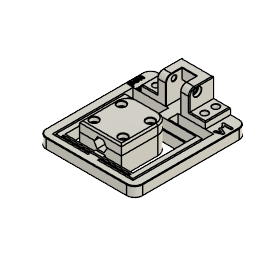
pen_mount (Autodesk Fusion 360 design; units mm, degrees)
Autodesk Fusion 360 part; units mm, degrees
sketch "Mount" plane through (0, 0, 0) normal (0, 0, 1) x (1, 0, 0) in component "Pen Mount"
  line L0 (30, -35) -> (-30, -35)
  line L1 (-30, -35) -> (-30, 35)
  line L2 (-30, 35) -> (30, 35)
  line L3 (30, 35) -> (30, -35)
  line L4 (30, -35) -> (-30, 35) construction
  line L5 (-30, -35) -> (30, 35) construction
  line L6 (25, 19) -> (25, -31)
  line L7 (-25, -31) -> (-25, 19)
  line L8 (0, 19) -> (0, -31) construction
  line L9 (0, 35) -> (0, -35) construction
  line L10 (24, 13) -> (24, -30)
  line L11 (-24, -30) -> (-24, 13)
  line L12 (-21, 12.2) -> (21, 12.2)
  line L13 (21, -29.2) -> (-21, -29.2)
  line L14 (-3, 13) -> (-3, 19)
  line L15 (3, 13) -> (3, 19)
  line L16 (-3, -30) -> (-3, -31)
  line L17 (3, -30) -> (3, -31)
  line L18 (24, -30) -> (3, -30)
  line L19 (-3, -30) -> (-24, -30)
  line L20 (-24, 13) -> (-3, 13)
  line L21 (3, 13) -> (24, 13)
  line L22 (-21, -27.2) -> (-3, -27.2)
  line L23 (-3, -27.2) -> (-3, -26.2)
  line L24 (-3, -26.2) -> (-13, -26.2)
  line L25 (-13, -26.2) -> (-13, -3.6)
  line L26 (-6, 3.4) -> (-3, 3.4)
  line L27 (-3, 3.4) -> (-3, 5.4)
  line L28 (-3, 5.4) -> (-21, 5.4)
  line L29 (-21, -28.2) -> (0, -28.2)
  line L30 (-21, 6.2) -> (0, 6.2)
  line L31 (-21, 6.2) -> (-21, 12.2)
  line L32 (-21, -29.2) -> (-21, -28.2)
  line L33 (-21, -27.2) -> (-21, 5.4)
  line L34 (21, 6.2) -> (21, 12.2)
  line L35 (21, 6.2) -> (0, 6.2)
  line L36 (3, 5.4) -> (21, 5.4)
  line L37 (3, 3.4) -> (3, 5.4)
  line L38 (6, 3.4) -> (3, 3.4)
  line L39 (13, -26.2) -> (13, -3.6)
  line L40 (21, -27.2) -> (21, 5.4)
  line L41 (3, -26.2) -> (13, -26.2)
  line L42 (3, -27.2) -> (3, -26.2)
  line L43 (21, -27.2) -> (3, -27.2)
  line L44 (21, -28.2) -> (0, -28.2)
  line L45 (21, -29.2) -> (21, -28.2)
  line L46 (-25, 19) -> (-3, 19)
  line L47 (3, 19) -> (25, 19)
  line L48 (25, -31) -> (3, -31)
  line L49 (-3, -31) -> (-25, -31)
  arc A0 (-6, 3.4) -> (-13, -3.6) centre (-6, -3.6) ccw
  arc A1 (13, -3.6) -> (6, 3.4) centre (6, -3.6) ccw
  circle A2 centre (-9, -4.2) radius 1.15
  circle A3 centre (-9, -21.2) radius 1.15
  line L50 (-9, -4.2) -> (-9, -21.2) construction
  circle A4 centre (9, -4.2) radius 1.15
  line L51 (9, -4.2) -> (9, -21.2) construction
  circle A5 centre (9, -21.2) radius 1.15
  circle A6 centre (-15, 30.5) radius 1.75
  line L52 (-15, 30.5) -> (-15, 23.5) construction
  circle A7 centre (-15, 23.5) radius 1.75
  circle A8 centre (15, 30.5) radius 1.75
  line L53 (15, 30.5) -> (15, 23.5) construction
  circle A9 centre (15, 23.5) radius 1.75
  line L54 (-4.2665, 3.4) -> (-4.2665, -26.2)
  line L55 (4.2665, 3.4) -> (4.2665, -26.2)
  line L56 (-3, 3.4) -> (3, 3.4)
  line L57 (-3, -26.2) -> (3, -26.2)
  dimension "d1" = 60
  dimension "d2" = 70
  dimension "d3" = 5
  dimension "d4" = 4
  dimension "d5" = 50
  dimension "d6" = 6
  dimension "d7" = 6
  dimension "d8" = 0.8
  dimension "d9" = 0.8
  dimension "d11" = 3
  dimension "d12" = 6
  dimension "d13" = 1
  dimension "d14" = 1
  dimension "d16" = 1
  dimension "d17" = 1
  dimension "d18" = 1
  dimension "d19" = 2
  dimension "d20" = 0.8
  dimension "d22" = 6
  dimension "d23" = 26
  dimension "d24" = 7
  dimension "d25" = 2.3
  dimension "d27" = 17
  dimension "d28" = 5
  dimension "d29" = 18
  dimension "d30" = 4
  dimension "d32" = 3.5
  dimension "d34" = 4.5
  dimension "d35" = 4.5
  dimension "d40" = 4.2665
  dimension "d73" = 30
  dimension "d74" = 7
  constraint horizontal L0
  constraint perpendicular L0 L1
  constraint parallel L0 L2
  constraint parallel L1 L3
  constraint coincident L4 origin
  constraint coincident L5 origin
  constraint horizontal L46
  constraint vertical L6
  constraint horizontal L48
  constraint vertical L7
  constraint midpoint L2 L9.start
  constraint midpoint L0 L9.end
  constraint collinear L8 L9
  constraint horizontal L20
  constraint vertical L10
  constraint horizontal L18
  constraint vertical L11
  constraint horizontal L12
  constraint horizontal L13
  constraint vertical L32
  constraint perpendicular L14 L46
  constraint symmetric L9 L14.start L15.start
  constraint symmetric L9 L14.end L15.end
  constraint coincident L16.start L18
  constraint coincident L16.end L48
  constraint perpendicular L16 L48
  constraint symmetric L9 L16.start L17.start
  constraint symmetric L9 L16.end L17.end
  constraint collinear L18 L19
  constraint collinear L20 L21
  constraint coincident L22.start L32
  constraint perpendicular L22 L32
  constraint perpendicular L22 L23
  constraint perpendicular L23 L24
  constraint perpendicular L24 L25
  constraint perpendicular L23 L26
  constraint perpendicular L26 L27
  constraint perpendicular L28 L32
  constraint horizontal L29
  constraint coincident L8 L29.end
  constraint coincident L9 L29.end
  constraint horizontal L30
  constraint coincident L30.start L32
  constraint coincident L8 L30.end
  constraint collinear L16 L23
  constraint collinear L14 L27
  constraint collinear L31 L32
  constraint collinear L32 L33
  constraint symmetric L8 L12.start L12.end
  constraint symmetric L8 L13.end L13.start
  constraint symmetric L8 L22.start L40.start
  constraint symmetric L8 L22.end L42.start
  constraint symmetric L8 L23.end L41.start
  constraint symmetric L8 L24.end L39.start
  constraint symmetric L8 L26.end L37.start
  constraint symmetric L8 L27.end L36.start
  constraint symmetric L8 L28.end L36.end
  constraint symmetric L8 L29.start L44.start
  constraint symmetric L8 L29.end L44.end
  constraint symmetric L8 L30.start L34.start
  constraint symmetric L8 L30.end L35.end
  constraint collinear L46 L47
  constraint coincident L8.start L46
  constraint collinear L48 L49
  constraint tangent L26 A0
  constraint tangent L25 A0
  constraint tangent L38 A1
  constraint tangent L39 A1
  constraint equal A0 A1
  constraint perpendicular L37 L38
  constraint equal A2 A3
  constraint coincident A2.centre L50.start
  constraint coincident A3.centre L50.end
  constraint vertical L50
  constraint symmetric L9 A2 A4
  constraint symmetric L9 A3 A5
  constraint symmetric L9 A2.centre A4.centre
  constraint symmetric L9 A3.centre L51.end
  constraint coincident L12.end L34.end
  constraint coincident L13.start L45.start
  constraint coincident A6.centre L52.start
  constraint vertical L52
  constraint coincident L52.end A7.centre
  constraint equal A6 A7
  constraint symmetric L9 A6 A8
  constraint symmetric L9 A6.centre A8.centre
  constraint symmetric L9 L52.end L53.end
  constraint symmetric L9 A7 A9
  constraint coincident L26 L54.start
  constraint coincident L24 L54.end
  constraint perpendicular L24 L54
  constraint symmetric L9 L54.start L55.start
  constraint symmetric L9 L54.end L55.end
  measures "d1" distance of L1.end L2.end
  measures "d2" distance of L0.end L1.end
  measures "d3" distance of L1 L7
  measures "d4" distance of L0 L48
  measures "d5" distance of L6.start L6.end
  measures "d6" distance of L14 L15
  measures "d7" distance of L16 L17
  measures "d8" distance of L12 L20
  measures "d9" distance of L13 L18
  measures "d11" distance of L11 L32
  measures "d12" distance of L14.start L14.end
  measures "d13" distance of L16.start L16.end
  measures "d14" distance of L7 L11
  measures "d16" distance of L13 L29
  measures "d17" distance of L22 L29
  measures "d18" distance of L22.end L23.end
  measures "d19" distance of L26.end L27.end
  measures "d20" distance of L28 L30
  measures "d22" distance of L12 L30
  measures "d23" distance of L25 L39
  measures "d24" radius of A0
  measures "d25" diameter of A2
  measures "d27" distance of A2.centre A3.centre
  measures "d28" distance of L24 A3.centre
  measures "d29" distance of L50 L51
  measures "d30" distance of L25 L50
  measures "d32" diameter of A6
  measures "d34" distance of L2 A6.centre
  measures "d35" distance of L46 L52.end
  measures "d40" distance of L9 L54
  measures "d73" distance of L52 L53
  measures "d74" distance of A6.centre L52.end
extrude "Extrude1" add sketch "Mount" along normal blind 6.5 contours L0 L1 L2 L3 | L24 L26 L38 L41 L54 L55 L56 L57 | L24 L25 L26 A0 L54 | L38 L39 L41 A1 L55 makes body 1 in component "Pen Mount"
extrude "Extrude3" add sketch "Mount" along normal blind 1 from surface at 6.5 contours L24 L26 L38 L41 L54 L55 L56 L57 | L24 L25 L26 A0 L54 | L38 L39 L41 A1 L55 bodies 1 in component "Pen Mount"
extrude "Extrude2" add sketch "Mount" along normal blind 3.695 from surface at 7.5 contours L24 L25 L26 A0 L54 | L38 L39 L41 A1 L55 bodies 1 in component "Pen Mount"
sketch "Sketch1" plane through (0, 0, 11.195) normal (0, 0, 1) x (-1, 0, 0) in component "Clamp"
  line L0 (4.2665, -3.4) -> (6, -3.4)
  arc A0 (6, -3.4) -> (13, 3.6) centre (6, 3.6) ccw
  line L1 (13, 3.6) -> (13, 26.2)
  line L2 (13, 26.2) -> (4.2665, 26.2)
  line L3 (4.2665, 26.2) -> (4.2665, -3.4)
  circle A1 centre (9, 4.2) radius 1.15
  circle A2 centre (9, 21.2) radius 1.15
  line L4 (4.2665, -3.4) -> (4.2665, 26.2)
  line L5 (4.2665, 26.2) -> (-4.2665, 26.2)
  line L6 (-4.2665, 26.2) -> (-4.2665, -3.4)
  line L7 (-4.2665, -3.4) -> (4.2665, -3.4)
  line L8 (-6, -3.4) -> (-4.2665, -3.4)
  line L9 (-4.2665, -3.4) -> (-4.2665, 26.2)
  line L10 (-4.2665, 26.2) -> (-13, 26.2)
  line L11 (-13, 26.2) -> (-13, 3.6)
  arc A3 (-13, 3.6) -> (-6, -3.4) centre (-6, 3.6) ccw
  circle A4 centre (-9, 4.2) radius 1.15
  circle A5 centre (-9, 21.2) radius 1.15
  line L12 (-3.6165, -3.4) -> (-3.6165, 26.2)
  line L13 (0, -3.4) -> (0, 26.2) construction
  line L14 (3.6165, -3.4) -> (3.6165, 26.2)
  circle A6 centre (9, 4.2) radius 1.48
  circle A7 centre (-9, 4.2) radius 1.48
  circle A8 centre (-9, 21.2) radius 1.48
  circle A9 centre (9, 21.2) radius 1.48
  dimension "d64" = 0.65
  dimension "d75" = 0.33
  constraint coincident L7 L12.start
  constraint coincident L5 L12.end
  constraint perpendicular L5 L12
  constraint midpoint L7 L13.start
  constraint midpoint L5 L13.end
  constraint symmetric L12.start L13 L14.start
  constraint symmetric L12.end L13 L14.end
  constraint concentric A4 A7
  constraint concentric A5 A8
  constraint concentric A2 A9
  constraint equal A6 A9
  constraint equal A6 A7
  constraint equal A6 A8
  measures "d64" distance of L6 L12
extrude "Extrude1'" add sketch "Sketch1" along normal blind 3 from surface at 2.995 separate body contours L5 L7 L12 L14 makes body 2 in component "Clamp"
extrude "Extrude2'" add sketch "Sketch1" along normal blind 5.995 contours L0 A0 L1 L2 L3 L4 | L3 L4 L5 L7 L14 | L5 L6 L7 L9 L12 | L6 L8 L9 L10 L11 A3 bodies 2 in component "Clamp"
draft "Draft1" angle 30 neutral plane through (0, 0, 11.195) pull (0, 0, -1) 1 faces at (3.6165, -6.4667, 12.1933) on bodies 2 in component "Clamp"
draft "Draft2" angle 30 neutral plane through (0, 0, 11.195) pull (0, 0, -1) 1 faces at (-3.6165, -6.4667, 12.1933) on bodies 2 in component "Clamp"
sketch "Sketch2" plane through (0, 0, 17.19) normal (0, 0, 1) x (-1, 0, 0) in component "Clamp"
  line L0 (13, 26.2) -> (-13, 26.2)
  line L1 (-6, -3.4) -> (6, -3.4)
  circle A0 centre (9, 21.2) radius 2.45
  circle A1 centre (9, 4.2) radius 2.45
  circle A2 centre (-9, 4.2) radius 2.45
  circle A3 centre (-9, 21.2) radius 2.45
  arc A4 (6, -3.4) -> (13, 3.6) centre (6, 3.6) ccw
  line L2 (13, 3.6) -> (13, 26.2)
  line L3 (-13, 26.2) -> (-13, 3.6)
  arc A5 (-13, 3.6) -> (-6, -3.4) centre (-6, 3.6) ccw
  circle A6 centre (9, 21.2) radius 1.48
  circle A7 centre (9, 4.2) radius 1.48
  circle A8 centre (-9, 21.2) radius 1.48
  circle A9 centre (-9, 4.2) radius 1.48
  dimension "d53" = 4.9
  constraint equal A0 A1
  constraint equal A0 A2
  constraint equal A0 A3
  constraint concentric A1 A7
  constraint concentric A2 A9
  constraint concentric A3 A8
  constraint concentric A0 A6
  measures "d53" diameter of A0
extrude "Extrude3'" cut sketch "Sketch2" against normal blind 2.65 contours A0 | A1 | A2 | A3 | A6 | A7 | A8 | A9 bodies 2 in component "Clamp"
chamfer "Chamfer1" distance 1 angle 45 6 edges at (0, 3.4, 17.19) (10.9497, 1.3497, 17.19) (13, -14.9, 17.19) (-13, -14.9, 17.19) (-10.9497, 1.3497, 17.19) (0, -26.2, 17.19) on bodies 2 in component "Clamp"
draft "Draft1'" angle 30 neutral plane through (0, 0, 11.195) pull (0, 0, 1) 1 faces at (-4.2665, -16.3333, 9.9633) on bodies 1 in component "Pen Mount"
draft "Draft2'" angle 30 neutral plane through (0, 0, 11.195) pull (0, 0, 1) 1 faces at (4.2665, -16.3333, 9.9633) on bodies 1 in component "Pen Mount"
fillet "Fillet1" radius 5 4 edges at (-30, -35, 3.25) (30, -35, 3.25) (30, 35, 3.25) (-30, 35, 3.25) on bodies 1 in component "Pen Mount"
chamfer "Chamfer1'" distance 0.3 angle 45 16 edges at (30, 0, 0) (28.5355, -33.5355, 0) (0, -35, 0) (-28.5355, -33.5355, 0) (-30, 0, 0) (-28.5355, 33.5355, 0) (0, 35, 0) (28.5355, 33.5355, 0) (30, 0, 6.5) (28.5355, 33.5355, 6.5) (0, 35, 6.5) (-28.5355, 33.5355, 6.5) (-30, 0, 6.5) (-28.5355, -33.5355, 6.5) (0, -35, 6.5) (28.5355, -33.5355, 6.5) on bodies 1 in component "Pen Mount"
sketch "Pen cross section" plane through (0, -26.2, 0) normal (0, -1, 0) x (1, 0, 0) in component "Pen Mount"
  line L0 (3, 0) -> (13, 0)
  line L1 (13, 0) -> (13, 11.195)
  line L2 (13, 11.195) -> (4.2665, 11.195)
  line L3 (4.2665, 11.195) -> (2.1332, 7.5)
  line L4 (2.1332, 7.5) -> (-2.1332, 7.5)
  line L5 (-2.1332, 7.5) -> (-4.2665, 11.195)
  line L6 (-4.2665, 11.195) -> (-13, 11.195)
  line L7 (-13, 11.195) -> (-13, 0)
  line L8 (-13, 0) -> (-3, 0)
  line L9 (-3, 0) -> (-3, 6.5)
  line L10 (-3, 6.5) -> (3, 6.5)
  line L11 (3, 6.5) -> (3, 0)
  line L12 (-2.1333, 7.5) -> (2.1333, 7.5)
  line L13 (2.1333, 7.5) -> (4.2666, 11.195)
  line L14 (4.2666, 11.195) -> (2.1333, 14.89)
  line L15 (2.1333, 14.89) -> (-2.1333, 14.89)
  line L16 (-2.1333, 14.89) -> (-4.2666, 11.195)
  line L17 (-4.2666, 11.195) -> (-2.1333, 7.5)
  line L18 (0, 14.89) -> (0, 7.5) construction
  point P0 (0, 11.195)
  dimension "d69" = 8.5332
  dimension "d70" = 7.39
  constraint collinear L4 L12
  constraint midpoint L15 L18.start
  constraint midpoint L12 L18.end
  constraint midpoint L4 L18.end
  measures "d69" distance of L13.end L16.end
  measures "d70" distance of L12 L15
fillet "Fillet1'" radius 0.5 2 edges at (-3.6165, -11.4, 11.195) (3.6165, -11.4, 11.195) on bodies 2 in component "Clamp"
sketch "Mounting screw heads" plane through (0, 0, 6.5) normal (0, 0, 1) x (-1, 0, 0) in component "Pen Mount"
  circle A0 centre (-15, -23.5) radius 1.75
  circle A1 centre (-15, -30.5) radius 1.75
  circle A2 centre (15, -23.5) radius 1.75
  circle A3 centre (15, -30.5) radius 1.75
  line L0 (-21, 29.2) -> (21, 29.2)
  line L1 (21, 29.2) -> (21, 28.2)
  line L2 (21, 28.2) -> (-21, 28.2)
  line L3 (-21, 28.2) -> (-21, 29.2)
  line L4 (-21, -6.2) -> (21, -6.2)
  line L5 (21, -6.2) -> (21, -12.2)
  line L6 (21, -12.2) -> (-21, -12.2)
  line L7 (-21, -12.2) -> (-21, -6.2)
  line L8 (24, 30) -> (3, 30)
  line L9 (3, 30) -> (3, 31)
  line L10 (3, 31) -> (25, 31)
  line L11 (25, 31) -> (25, -19)
  line L12 (25, -19) -> (3, -19)
  line L13 (3, -19) -> (3, -13)
  line L14 (3, -13) -> (24, -13)
  line L15 (24, -13) -> (24, 30)
  line L16 (-3, 26.2) -> (3, 26.2)
  line L17 (3, 26.2) -> (3, 27.2)
  line L18 (3, 27.2) -> (21, 27.2)
  line L19 (21, 27.2) -> (21, -5.4)
  line L20 (21, -5.4) -> (3, -5.4)
  line L21 (3, -5.4) -> (3, -3.4)
  line L22 (3, -3.4) -> (-3, -3.4)
  line L23 (-3, -3.4) -> (-3, -5.4)
  line L24 (-3, -5.4) -> (-21, -5.4)
  line L25 (-21, -5.4) -> (-21, 27.2)
  line L26 (-21, 27.2) -> (-3, 27.2)
  line L27 (-3, 27.2) -> (-3, 26.2)
  line L28 (-24, -13) -> (-3, -13)
  line L29 (-3, -13) -> (-3, -19)
  line L30 (-3, -19) -> (-25, -19)
  line L31 (-25, -19) -> (-25, 31)
  line L32 (-25, 31) -> (-3, 31)
  line L33 (-3, 31) -> (-3, 30)
  line L34 (-3, 30) -> (-24, 30)
  line L35 (-24, 30) -> (-24, -13)
  line L36 (29.7, -30) -> (29.7, 30)
  arc A4 (29.7, 30) -> (25, 34.7) centre (25, 30) ccw
  line L37 (25, 34.7) -> (-25, 34.7)
  arc A5 (-25, 34.7) -> (-29.7, 30) centre (-25, 30) ccw
  line L38 (-29.7, 30) -> (-29.7, -30)
  arc A6 (-29.7, -30) -> (-25, -34.7) centre (-25, -30) ccw
  line L39 (-25, -34.7) -> (25, -34.7)
  arc A7 (25, -34.7) -> (29.7, -30) centre (25, -30) ccw
  circle A8 centre (15, -30.5) radius 3
  circle A9 centre (15, -23.5) radius 3
  circle A10 centre (-15, -30.5) radius 3
  circle A11 centre (-15, -23.5) radius 3
  line L40 (-27.7, -20) -> (-27.7, -33.2) construction
  line L41 (-27.7, -33.2) -> (-22.2993, -33.2) construction
  line L42 (-22.2993, -33.2) -> (-22.2993, -20) construction
  line L43 (-22.2993, -20) -> (-27.7, -20) construction
  line L44 (24.0828, -19.2154) -> (24.0761, -31.7956) construction
  line L45 (24.0761, -31.7956) -> (29.0761, -31.7983) construction
  line L46 (29.0761, -31.7983) -> (29.0828, -19.2181) construction
  line L47 (29.0828, -19.2181) -> (24.0828, -19.2154) construction
  dimension "d76" = 6
  dimension "d87" = 6
  dimension "d88" = 1
  dimension "d89" = 1.5
  dimension "d90" = 2
  dimension "d93" = 3.7
  text T0 "v1\n" font "Arial" height 6 bold align left top in box 13.2 x 5.4007 at (-27.7, -20) x (0, -1) y (1, 0) spacing 1 kerned
  text T1 "pen\nmount" font "Arial" height 3.7 bold align left top in box 12.5802 x 5 at (24.0828, -19.2154) x (-0.000531, -1) y (1, -0.000531) spacing 1 kerned
  constraint concentric A3 A8
  constraint concentric A2 A9
  constraint concentric A1 A10
  constraint concentric A0 A11
  constraint equal A8 A9
  constraint equal A8 A10
  constraint equal A8 A11
  measures "d76" diameter of A8
  measures "d88" distance of L30 L43
  measures "d89" distance of L39 L41
  measures "d90" distance of L38 L40
fillet "Fillet2" radius 0.25 4 faces at (-13.2587, 23.3258, 4.3333) (-13.2587, 30.3258, 4.3333) (16.7413, 30.3258, 4.3333) (16.7413, 23.3258, 4.3333) on bodies 1 in component "Pen Mount"
fillet "Fillet2" radius 0.25 4 faces at (-7.8557, -4.3145, 3.7317) (-8.3287, -20.2663, 3.7317) (10.1443, -4.3145, 3.7317) (9.6713, -20.2663, 3.7317) on bodies 1 in component "Pen Mount"
fillet "Fillet2'" radius 0.25 4 edges at (-6.7158, -5.086, 17.19) (11.2842, -5.086, 17.19) (11.2842, -22.086, 17.19) (-6.7158, -22.086, 17.19) on bodies 2 in component "Clamp"
extrude "Extrude4" add sketch "Mounting screw heads" along normal blind 0.2 text T0 T1 bodies 1 in component "Pen Mount"
sketch "Sketch1 (2)" plane through (0, 0, 6.5) normal (0, 0, 1) x (-1, 0, 0) in component "Weight mount"
  spline S0 degree 3 poles (21.9429, -23.6992) (22.0605, -23.7069) (22.2992, -23.7226) (22.5165, -23.8229) (22.6268, -23.8737) knots 0 0 0 0 0.035038 0.071116 0.071116 0.071116 0.071116
  spline S1 degree 3 poles (22.6268, -23.8737) (22.7302, -23.9375) (22.9356, -24.0641) (23.0664, -24.2668) (23.1313, -24.3674) knots 0 0 0 0 0.035952 0.071388 0.071388 0.071388 0.071388
  spline S2 degree 3 poles (23.1313, -24.3674) (23.182, -24.4783) (23.2856, -24.7047) (23.2985, -24.9535) (23.3051, -25.0805) knots 0 0 0 0 0.036225 0.073988 0.073988 0.073988 0.073988
  spline S3 degree 3 poles (23.3051, -25.0805) (23.2903, -25.2723) (23.2615, -25.6461) (23.0248, -25.936) (22.9095, -26.0772) knots 0 0 0 0 0.05621 0.10955 0.10955 0.10955 0.10955
  spline S4 degree 3 poles (22.9095, -26.0772) (22.7669, -26.1905) (22.4745, -26.4225) (22.1019, -26.4509) (21.9111, -26.4654) knots 0 0 0 0 0.053369 0.109334 0.109334 0.109334 0.109334
  spline S5 degree 3 poles (21.9111, -26.4654) (21.7187, -26.4505) (21.3424, -26.4213) (21.0473, -26.1869) (20.9031, -26.0724) knots 0 0 0 0 0.056479 0.110425 0.110425 0.110425 0.110425
  spline S6 degree 3 poles (20.9031, -26.0724) (20.7865, -25.9314) (20.5492, -25.6444) (20.5189, -25.273) (20.5036, -25.0841) knots 0 0 0 0 0.053525 0.108919 0.108919 0.108919 0.108919
  spline S7 degree 3 poles (20.5036, -25.0841) (20.5107, -24.9625) (20.5249, -24.7184) (20.6219, -24.4939) (20.6705, -24.3812) knots 0 0 0 0 0.036237 0.072735 0.072735 0.072735 0.072735
  spline S8 degree 3 poles (20.6705, -24.3812) (20.7322, -24.2766) (20.8551, -24.0686) (21.0582, -23.9379) (21.1591, -23.8729) knots 0 0 0 0 0.035892 0.071384 0.071384 0.071384 0.071384
  spline S9 degree 3 poles (21.1591, -23.8729) (21.2764, -23.8223) (21.5262, -23.7144) (21.7985, -23.7045) (21.9429, -23.6992) knots 0 0 0 0 0.037997 0.080903 0.080903 0.080903 0.080903
  line L0 (23.2476, -19.215) -> (23.2473, -19.8687)
  line L1 (23.2473, -19.8687) -> (22.8813, -19.8685)
  spline S10 degree 3 poles (22.8813, -19.8685) (23.0056, -19.9878) (23.2451, -20.2177) (23.2872, -20.5461) (23.3074, -20.7041) knots 0 0 0 0 0.049999 0.096357 0.096357 0.096357 0.096357
  spline S11 degree 3 poles (23.3074, -20.7041) (23.3038, -20.7855) (23.2969, -20.9414) (23.2321, -21.0831) (23.2011, -21.1508) knots 0 0 0 0 0.024186 0.046297 0.046297 0.046297 0.046297
  spline S12 degree 3 poles (23.2011, -21.1508) (23.1601, -21.2116) (23.0752, -21.3376) (22.9468, -21.419) (22.8804, -21.461) knots 0 0 0 0 0.021771 0.045054 0.045054 0.045054 0.045054
  spline S13 degree 3 poles (22.8804, -21.461) (22.9464, -21.5193) (23.0723, -21.6305) (23.1594, -21.774) (23.2008, -21.8423) knots 0 0 0 0 0.026236 0.050053 0.050053 0.050053 0.050053
  spline S14 degree 3 poles (23.2008, -21.8423) (23.2317, -21.9117) (23.2935, -22.0508) (23.3022, -22.2028) (23.3065, -22.279) knots 0 0 0 0 0.022583 0.045264 0.045264 0.045264 0.045264
  spline S15 degree 3 poles (23.3065, -22.279) (23.3028, -22.3714) (23.2956, -22.5461) (23.2214, -22.7042) (23.1864, -22.7787) knots 0 0 0 0 0.027422 0.051852 0.051852 0.051852 0.051852
  spline S16 degree 3 poles (23.1864, -22.7787) (23.1411, -22.8428) (23.0487, -22.9733) (22.9065, -23.0466) (22.8342, -23.0839) knots 0 0 0 0 0.02319 0.047221 0.047221 0.047221 0.047221
  spline S17 degree 3 poles (22.8342, -23.0839) (22.7597, -23.105) (22.5786, -23.1564) (22.3899, -23.1566) (22.2789, -23.1568) knots 0 0 0 0 0.023124 0.056237 0.056237 0.056237 0.056237
  line L2 (22.2789, -23.1568) -> (20.5652, -23.1558)
  line L3 (20.5652, -23.1558) -> (20.5655, -22.4466)
  line L4 (20.5655, -22.4466) -> (22.0975, -22.4475)
  spline S18 degree 3 poles (22.0975, -22.4475) (22.2082, -22.4492) (22.3845, -22.452) (22.5506, -22.3955) (22.6124, -22.3745) knots 0 0 0 0 0.032861 0.052328 0.052328 0.052328 0.052328
  spline S19 degree 3 poles (22.6124, -22.3745) (22.6566, -22.3361) (22.7484, -22.2564) (22.7587, -22.1348) (22.764, -22.0717) knots 0 0 0 0 0.016884 0.035076 0.035076 0.035076 0.035076
  spline S20 degree 3 poles (22.764, -22.0717) (22.76, -22.0225) (22.7518, -21.922) (22.6998, -21.8356) (22.6733, -21.7915) knots 0 0 0 0 0.014627 0.029808 0.029808 0.029808 0.029808
  spline S21 degree 3 poles (22.6733, -21.7915) (22.6384, -21.7505) (22.5659, -21.665) (22.4614, -21.6236) (22.4071, -21.6021) knots 0 0 0 0 0.015906 0.033119 0.033119 0.033119 0.033119
  spline S22 degree 3 poles (22.4071, -21.6021) (22.332, -21.5853) (22.1499, -21.5444) (21.963, -21.544) (21.8532, -21.5438) knots 0 0 0 0 0.023035 0.055846 0.055846 0.055846 0.055846
  line L5 (21.8532, -21.5438) -> (20.566, -21.5431)
  line L6 (20.566, -21.5431) -> (20.5664, -20.8339)
  line L7 (20.5664, -20.8339) -> (22.0353, -20.8347)
  spline S23 degree 3 poles (22.0353, -20.8347) (22.1429, -20.8358) (22.3125, -20.8376) (22.4792, -20.8079) (22.5401, -20.7971) knots 0 0 0 0 0.032193 0.05071 0.05071 0.05071 0.05071
  spline S24 degree 3 poles (22.5401, -20.7971) (22.5749, -20.7836) (22.6409, -20.758) (22.6873, -20.7049) (22.7092, -20.6798) knots 0 0 0 0 0.01102 0.020858 0.020858 0.020858 0.020858
  spline S25 degree 3 poles (22.7092, -20.6798) (22.7254, -20.6492) (22.761, -20.5819) (22.7635, -20.5056) (22.7649, -20.464) knots 0 0 0 0 0.010254 0.022541 0.022541 0.022541 0.022541
  spline S26 degree 3 poles (22.7649, -20.464) (22.7614, -20.4109) (22.7544, -20.3058) (22.7024, -20.2141) (22.6767, -20.1687) knots 0 0 0 0 0.015741 0.031179 0.031179 0.031179 0.031179
  spline S27 degree 3 poles (22.6767, -20.1687) (22.6433, -20.1278) (22.5744, -20.0435) (22.4737, -20.0019) (22.4219, -19.9805) knots 0 0 0 0 0.015597 0.032119 0.032119 0.032119 0.032119
  spline S28 degree 3 poles (22.4219, -19.9805) (22.3483, -19.9641) (22.1666, -19.9234) (21.9802, -19.9234) (21.8692, -19.9235) knots 0 0 0 0 0.022553 0.055709 0.055709 0.055709 0.055709
  line L8 (21.8692, -19.9235) -> (20.5669, -19.9228)
  line L9 (20.5669, -19.9228) -> (20.5672, -19.2136)
  line L10 (20.5672, -19.2136) -> (23.2476, -19.215)
  circle A0 centre (-15, -23.5) radius 2
  circle A1 centre (15, -30.5) radius 2
  line L11 (-29.7, 30) -> (-29.7, -30)
  arc A2 (-29.7, -30) -> (-25, -34.7) centre (-25, -30) ccw
  line L12 (-25, -34.7) -> (25, -34.7)
  arc A3 (25, -34.7) -> (29.7, -30) centre (25, -30) ccw
  line L13 (29.7, -30) -> (29.7, 30)
  arc A4 (29.7, 30) -> (25, 34.7) centre (25, 30) ccw
  line L14 (25, 34.7) -> (-25, 34.7)
  arc A5 (-25, 34.7) -> (-29.7, 30) centre (-25, 30) ccw
  line L15 (-21, -6.2) -> (21, -6.2)
  line L16 (21, -6.2) -> (21, -12.2)
  line L17 (21, -12.2) -> (-21, -12.2)
  line L18 (-21, -12.2) -> (-21, -6.2)
  line L19 (-21, 29.2) -> (21, 29.2)
  line L20 (21, 29.2) -> (21, 28.2)
  line L21 (21, 28.2) -> (-21, 28.2)
  line L22 (-21, 28.2) -> (-21, 29.2)
  line L23 (-24, -13) -> (-3, -13)
  line L24 (-3, -13) -> (-3, -19)
  line L25 (-3, -19) -> (-25, -19)
  line L26 (-25, -19) -> (-25, 31)
  line L27 (-25, 31) -> (-3, 31)
  line L28 (-3, 31) -> (-3, 30)
  line L29 (-3, 30) -> (-24, 30)
  line L30 (-24, 30) -> (-24, -13)
  line L31 (24, 30) -> (3, 30)
  line L32 (3, 30) -> (3, 31)
  line L33 (3, 31) -> (25, 31)
  line L34 (25, 31) -> (25, -19)
  line L35 (25, -19) -> (3, -19)
  line L36 (3, -19) -> (3, -13)
  line L37 (3, -13) -> (24, -13)
  line L38 (24, -13) -> (24, 30)
  line L39 (-3, 26.2) -> (3, 26.2)
  line L40 (3, 26.2) -> (3, 27.2)
  line L41 (3, 27.2) -> (21, 27.2)
  line L42 (21, 27.2) -> (21, -5.4)
  line L43 (21, -5.4) -> (3, -5.4)
  line L44 (3, -5.4) -> (3, -3.4)
  line L45 (3, -3.4) -> (-3, -3.4)
  line L46 (-3, -3.4) -> (-3, -5.4)
  line L47 (-3, -5.4) -> (-21, -5.4)
  line L48 (-21, -5.4) -> (-21, 27.2)
  line L49 (-21, 27.2) -> (-3, 27.2)
  line L50 (-3, 27.2) -> (-3, 26.2)
  circle A6 centre (15, -23.5) radius 2
  circle A7 centre (-15, -30.5) radius 2
  line L51 (27.1924, -23.9796) -> (27.0734, -24.6862)
  spline S29 degree 3 poles (27.0734, -24.6862) (26.953, -24.6362) (26.7211, -24.5397) (26.5595, -24.3479) (26.4818, -24.2556) knots 0 0 0 0 0.038477 0.074127 0.074127 0.074127 0.074127
  spline S30 degree 3 poles (26.4818, -24.2556) (26.4226, -24.1477) (26.2973, -23.9189) (26.2853, -23.6577) (26.279, -23.5198) knots 0 0 0 0 0.036434 0.077228 0.077228 0.077228 0.077228
  spline S31 degree 3 poles (26.279, -23.5198) (26.293, -23.3059) (26.3194, -22.903) (26.6032, -22.6187) (26.7364, -22.4852) knots 0 0 0 0 0.061888 0.116598 0.116598 0.116598 0.116598
  spline S32 degree 3 poles (26.7364, -22.4852) (26.8711, -22.4081) (27.1568, -22.2445) (27.4862, -22.229) (27.6603, -22.2207) knots 0 0 0 0 0.045916 0.097327 0.097327 0.097327 0.097327
  spline S33 degree 3 poles (27.6603, -22.2207) (27.865, -22.2307) (28.2469, -22.2493) (28.5589, -22.4681) (28.7037, -22.5696) knots 0 0 0 0 0.06004 0.112035 0.112035 0.112035 0.112035
  spline S34 degree 3 poles (28.7037, -22.5696) (28.8137, -22.6943) (29.0359, -22.9464) (29.0656, -23.2814) (29.0805, -23.4506) knots 0 0 0 0 0.048539 0.098092 0.098092 0.098092 0.098092
  spline S35 degree 3 poles (29.0805, -23.4506) (29.0666, -23.6371) (29.0397, -23.9967) (28.8003, -24.2651) (28.6851, -24.3943) knots 0 0 0 0 0.05441 0.1049 0.1049 0.1049 0.1049
  spline S36 degree 3 poles (28.6851, -24.3943) (28.5226, -24.4938) (28.1536, -24.7199) (27.7183, -24.7227) (27.4747, -24.7243) knots 0 0 0 0 0.056156 0.127567 0.127567 0.127567 0.127567
  line L52 (27.4747, -24.7243) -> (27.4756, -22.9475)
  spline S37 degree 3 poles (27.4756, -22.9475) (27.3789, -22.9542) (27.199, -22.9667) (27.0524, -23.0707) (26.9846, -23.1189) knots 0 0 0 0 0.028433 0.052905 0.052905 0.052905 0.052905
  spline S38 degree 3 poles (26.9846, -23.1189) (26.9335, -23.1771) (26.8305, -23.2942) (26.8162, -23.4496) (26.809, -23.5276) knots 0 0 0 0 0.022639 0.045526 0.045526 0.045526 0.045526
  spline S39 degree 3 poles (26.809, -23.5276) (26.8122, -23.5802) (26.8183, -23.6816) (26.8733, -23.7668) (26.8997, -23.8078) knots 0 0 0 0 0.0155 0.029897 0.029897 0.029897 0.029897
  spline S40 degree 3 poles (26.8997, -23.8078) (26.9374, -23.8441) (27.0209, -23.9246) (27.1316, -23.9601) (27.1924, -23.9796) knots 0 0 0 0 0.015495 0.034337 0.034337 0.034337 0.034337
  line L53 (20.5601, -32.6153) -> (20.5605, -31.9061)
  line L54 (20.5605, -31.9061) -> (21.9284, -31.9068)
  spline S41 degree 3 poles (21.9284, -31.9068) (22.0481, -31.9081) (22.237, -31.9102) (22.4222, -31.8747) (22.49, -31.8617) knots 0 0 0 0 0.035762 0.056457 0.056457 0.056457 0.056457
  spline S42 degree 3 poles (22.49, -31.8617) (22.5299, -31.8446) (22.6078, -31.8112) (22.6618, -31.746) (22.6882, -31.7142) knots 0 0 0 0 0.0128 0.025026 0.025026 0.025026 0.025026
  spline S43 degree 3 poles (22.6882, -31.7142) (22.7089, -31.6775) (22.7518, -31.6012) (22.7566, -31.5136) (22.759, -31.4681) knots 0 0 0 0 0.012448 0.025909 0.025909 0.025909 0.025909
  spline S44 degree 3 poles (22.759, -31.4681) (22.755, -31.4085) (22.7471, -31.2904) (22.6877, -31.1881) (22.6583, -31.1375) knots 0 0 0 0 0.017659 0.034986 0.034986 0.034986 0.034986
  spline S45 degree 3 poles (22.6583, -31.1375) (22.622, -31.0925) (22.5498, -31.003) (22.4437, -30.9587) (22.3908, -30.9367) knots 0 0 0 0 0.017026 0.033916 0.033916 0.033916 0.033916
  spline S46 degree 3 poles (22.3908, -30.9367) (22.312, -30.921) (22.109, -30.8806) (21.9018, -30.8815) (21.775, -30.8821) knots 0 0 0 0 0.024071 0.061953 0.061953 0.061953 0.061953
  line L55 (21.775, -30.8821) -> (20.5611, -30.8814)
  line L56 (20.5611, -30.8814) -> (20.5614, -30.1722)
  line L57 (20.5614, -30.1722) -> (23.2418, -30.1736)
  line L58 (23.2418, -30.1736) -> (23.2414, -30.8324)
  line L59 (23.2414, -30.8324) -> (22.8477, -30.8322)
  spline S47 degree 3 poles (22.8477, -30.8322) (22.9801, -30.9547) (23.2393, -31.1946) (23.2811, -31.5446) (23.3015, -31.7158) knots 0 0 0 0 0.052259 0.102277 0.102277 0.102277 0.102277
  spline S48 degree 3 poles (23.3015, -31.7158) (23.2984, -31.7914) (23.2922, -31.9388) (23.2414, -32.0773) (23.2168, -32.1448) knots 0 0 0 0 0.022562 0.043966 0.043966 0.043966 0.043966
  spline S49 degree 3 poles (23.2168, -32.1448) (23.1882, -32.2043) (23.1347, -32.3161) (23.0434, -32.3996) (23.0008, -32.4387) knots 0 0 0 0 0.019593 0.036773 0.036773 0.036773 0.036773
  spline S50 degree 3 poles (23.0008, -32.4387) (22.9553, -32.4694) (22.8634, -32.5315) (22.7568, -32.562) (22.7029, -32.5773) knots 0 0 0 0 0.016361 0.033043 0.033043 0.033043 0.033043
  spline S51 degree 3 poles (22.7029, -32.5773) (22.6355, -32.5887) (22.4777, -32.6152) (22.3176, -32.6158) (22.2259, -32.6162) knots 0 0 0 0 0.020465 0.04793 0.04793 0.04793 0.04793
  line L60 (22.2259, -32.6162) -> (20.5601, -32.6153)
  line L61 (-28.2993, -27.9154) -> (-28.2993, -26.7653)
  line L62 (-28.2993, -26.7653) -> (-23.965, -26.7653)
  spline S52 degree 3 poles (-23.965, -26.7653) (-24.1492, -26.5443) (-24.5217, -26.0973) (-24.731, -25.5542) (-24.8368, -25.2797) knots 0 0 0 0 0.085682 0.173293 0.173293 0.173293 0.173293
  line L63 (-24.8368, -25.2797) -> (-23.7931, -25.2797)
  spline S53 degree 3 poles (-23.7931, -25.2797) (-23.7278, -25.4395) (-23.5847, -25.7897) (-23.3578, -26.093) (-23.2345, -26.2578) knots 0 0 0 0 0.051583 0.113052 0.113052 0.113052 0.113052
  spline S54 degree 3 poles (-23.2345, -26.2578) (-23.0952, -26.4187) (-22.8267, -26.729) (-22.4541, -26.8999) (-22.2747, -26.9823) knots 0 0 0 0 0.062981 0.121495 0.121495 0.121495 0.121495
  line L64 (-22.2747, -26.9823) -> (-22.2747, -27.9154)
  line L65 (-22.2747, -27.9154) -> (-28.2993, -27.9154)
  line L66 (-28.2993, -21.7517) -> (-23.9527, -20)
  line L67 (-23.9527, -20) -> (-23.9527, -21.2074)
  line L68 (-23.9527, -21.2074) -> (-26.171, -22.0259)
  line L69 (-26.171, -22.0259) -> (-26.9118, -22.2633)
  spline S55 degree 3 poles (-26.9118, -22.2633) (-26.8339, -22.2894) (-26.7103, -22.3308) (-26.5855, -22.3682) (-26.5394, -22.382) knots 0 0 0 0 0.024656 0.039092 0.039092 0.039092 0.039092
  spline S56 degree 3 poles (-26.5394, -22.382) (-26.4779, -22.4015) (-26.3545, -22.4406) (-26.2323, -22.4833) (-26.171, -22.5048) knots 0 0 0 0 0.01935 0.038829 0.038829 0.038829 0.038829
  line L70 (-26.171, -22.5048) -> (-23.9527, -23.3315)
  line L71 (-23.9527, -23.3315) -> (-23.9527, -24.5143)
  line L72 (-23.9527, -24.5143) -> (-28.2993, -22.7872)
  line L73 (-28.2993, -22.7872) -> (-28.2993, -21.7517)
  line L74 (20.5622, -28.7841) -> (20.9635, -28.7843)
  spline S57 degree 3 poles (20.9635, -28.7843) (20.8956, -28.7313) (20.7586, -28.6243) (20.6701, -28.4747) (20.6255, -28.3992) knots 0 0 0 0 0.025592 0.051642 0.051642 0.051642 0.051642
  spline S58 degree 3 poles (20.6255, -28.3992) (20.5894, -28.3188) (20.5176, -28.1584) (20.5072, -27.983) (20.5021, -27.8957) knots 0 0 0 0 0.026209 0.052232 0.052232 0.052232 0.052232
  spline S59 degree 3 poles (20.5021, -27.8957) (20.5065, -27.8089) (20.5152, -27.6397) (20.5863, -27.486) (20.6209, -27.4111) knots 0 0 0 0 0.025788 0.050301 0.050301 0.050301 0.050301
  spline S60 degree 3 poles (20.6209, -27.4111) (20.6641, -27.3448) (20.7494, -27.2136) (20.8865, -27.1381) (20.9543, -27.1009) knots 0 0 0 0 0.023348 0.046168 0.046168 0.046168 0.046168
  spline S61 degree 3 poles (20.9543, -27.1009) (21.0388, -27.073) (21.231, -27.0098) (21.4338, -27.0069) (21.5474, -27.0053) knots 0 0 0 0 0.026547 0.060389 0.060389 0.060389 0.060389
  line L75 (21.5474, -27.0053) -> (23.2435, -27.0062)
  line L76 (23.2435, -27.0062) -> (23.2431, -27.7154)
  line L77 (23.2431, -27.7154) -> (22.0114, -27.7147)
  spline S62 degree 3 poles (22.0114, -27.7147) (21.8591, -27.7129) (21.627, -27.71) (21.3975, -27.7424) (21.3186, -27.7535) knots 0 0 0 0 0.045598 0.069472 0.069472 0.069472 0.069472
  spline S63 degree 3 poles (21.3186, -27.7535) (21.2785, -27.769) (21.1992, -27.7996) (21.1439, -27.8641) (21.1166, -27.896) knots 0 0 0 0 0.012685 0.025066 0.025066 0.025066 0.025066
  spline S64 degree 3 poles (21.1166, -27.896) (21.0949, -27.9342) (21.0487, -28.0154) (21.0444, -28.1089) (21.042, -28.1584) knots 0 0 0 0 0.012997 0.027628 0.027628 0.027628 0.027628
  spline S65 degree 3 poles (21.042, -28.1584) (21.046, -28.2172) (21.0538, -28.3335) (21.1125, -28.4342) (21.1416, -28.4841) knots 0 0 0 0 0.017405 0.034463 0.034463 0.034463 0.034463
  spline S66 degree 3 poles (21.1416, -28.4841) (21.176, -28.528) (21.2429, -28.6133) (21.3411, -28.6589) (21.3888, -28.681) knots 0 0 0 0 0.016477 0.032013 0.032013 0.032013 0.032013
  spline S67 degree 3 poles (21.3888, -28.681) (21.4735, -28.6963) (21.7122, -28.7392) (21.9551, -28.7363) (22.1118, -28.7344) knots 0 0 0 0 0.025768 0.072636 0.072636 0.072636 0.072636
  line L78 (22.1118, -28.7344) -> (23.2425, -28.735)
  line L79 (23.2425, -28.735) -> (23.2422, -29.4442)
  line L80 (23.2422, -29.4442) -> (20.5618, -29.4428)
  line L81 (20.5618, -29.4428) -> (20.5622, -28.7841)
  line L82 (23.2395, -34.5652) -> (22.6741, -34.5649)
  line L83 (22.6741, -34.5649) -> (22.6744, -34.0803)
  line L84 (22.6744, -34.0803) -> (21.5941, -34.0797)
  spline S68 degree 3 poles (21.5941, -34.0797) (21.5075, -34.0787) (21.3797, -34.0773) (21.2527, -34.0895) (21.2118, -34.0934) knots 0 0 0 0 0.025967 0.038283 0.038283 0.038283 0.038283
  spline S69 degree 3 poles (21.2118, -34.0934) (21.1943, -34.0997) (21.1587, -34.1125) (21.1345, -34.1416) (21.1221, -34.1565) knots 0 0 0 0 0.005449 0.011138 0.011138 0.011138 0.011138
  spline S70 degree 3 poles (21.1221, -34.1565) (21.1118, -34.1742) (21.0903, -34.2112) (21.088, -34.254) (21.0867, -34.2763) knots 0 0 0 0 0.006067 0.012657 0.012657 0.012657 0.012657
  spline S71 degree 3 poles (21.0867, -34.2763) (21.0911, -34.3168) (21.1016, -34.4146) (21.1351, -34.5072) (21.1547, -34.5616) knots 0 0 0 0 0.012171 0.029414 0.029414 0.029414 0.029414
  line L85 (21.1547, -34.5616) -> (20.6045, -34.6218)
  spline S72 degree 3 poles (20.6045, -34.6218) (20.5736, -34.5348) (20.5094, -34.3536) (20.5024, -34.1613) (20.4988, -34.0615) knots 0 0 0 0 0.027547 0.05732 0.05732 0.05732 0.05732
  spline S73 degree 3 poles (20.4988, -34.0615) (20.5011, -34.0001) (20.5056, -33.8816) (20.5445, -33.7697) (20.5633, -33.7157) knots 0 0 0 0 0.018306 0.035346 0.035346 0.035346 0.035346
  spline S74 degree 3 poles (20.5633, -33.7157) (20.5849, -33.669) (20.625, -33.582) (20.6968, -33.519) (20.73, -33.4899) knots 0 0 0 0 0.015251 0.028346 0.028346 0.028346 0.028346
  spline S75 degree 3 poles (20.73, -33.4899) (20.7693, -33.4675) (20.8555, -33.4183) (20.9532, -33.4002) (21.0064, -33.3904) knots 0 0 0 0 0.013474 0.029565 0.029565 0.029565 0.029565
  spline S76 degree 3 poles (21.0064, -33.3904) (21.0687, -33.3839) (21.2347, -33.3666) (21.4017, -33.3674) (21.5062, -33.3679) knots 0 0 0 0 0.018754 0.050055 0.050055 0.050055 0.050055
  line L86 (21.5062, -33.3679) -> (22.6747, -33.3686)
  line L87 (22.6747, -33.3686) -> (22.6749, -33.043)
  line L88 (22.6749, -33.043) -> (23.2403, -33.0433)
  line L89 (23.2403, -33.0433) -> (23.2401, -33.3689)
  line L90 (23.2401, -33.3689) -> (23.7726, -33.3691)
  line L91 (23.7726, -33.3691) -> (24.1862, -34.0811)
  line L92 (24.1862, -34.0811) -> (23.2397, -34.0806)
  line L93 (23.2397, -34.0806) -> (23.2395, -34.5652)
  line L94 (26.3373, -27.7397) -> (26.3377, -27.0305)
  line L95 (26.3377, -27.0305) -> (27.7057, -27.0313)
  spline S77 degree 3 poles (27.7057, -27.0313) (27.8253, -27.0326) (28.0142, -27.0346) (28.1994, -26.9991) (28.2672, -26.9861) knots 0 0 0 0 0.035762 0.056457 0.056457 0.056457 0.056457
  spline S78 degree 3 poles (28.2672, -26.9861) (28.3071, -26.969) (28.385, -26.9356) (28.439, -26.8704) (28.4654, -26.8386) knots 0 0 0 0 0.0128 0.025026 0.025026 0.025026 0.025026
  spline S79 degree 3 poles (28.4654, -26.8386) (28.4861, -26.8019) (28.529, -26.7256) (28.5338, -26.638) (28.5362, -26.5925) knots 0 0 0 0 0.012448 0.025909 0.025909 0.025909 0.025909
  spline S80 degree 3 poles (28.5362, -26.5925) (28.5322, -26.5329) (28.5243, -26.4149) (28.4649, -26.3125) (28.4355, -26.2619) knots 0 0 0 0 0.017659 0.034986 0.034986 0.034986 0.034986
  spline S81 degree 3 poles (28.4355, -26.2619) (28.3992, -26.2169) (28.327, -26.1274) (28.2209, -26.0831) (28.168, -26.0611) knots 0 0 0 0 0.017026 0.033916 0.033916 0.033916 0.033916
  spline S82 degree 3 poles (28.168, -26.0611) (28.0892, -26.0454) (27.8862, -26.005) (27.679, -26.0059) (27.5522, -26.0065) knots 0 0 0 0 0.024071 0.061953 0.061953 0.061953 0.061953
  line L96 (27.5522, -26.0065) -> (26.3383, -26.0058)
  line L97 (26.3383, -26.0058) -> (26.3386, -25.2966)
  line L98 (26.3386, -25.2966) -> (29.019, -25.2981)
  line L99 (29.019, -25.2981) -> (29.0186, -25.9568)
  line L100 (29.0186, -25.9568) -> (28.6249, -25.9566)
  spline S83 degree 3 poles (28.6249, -25.9566) (28.7573, -26.0791) (29.0165, -26.319) (29.0583, -26.669) (29.0787, -26.8402) knots 0 0 0 0 0.052259 0.102277 0.102277 0.102277 0.102277
  spline S84 degree 3 poles (29.0787, -26.8402) (29.0756, -26.9158) (29.0694, -27.0633) (29.0187, -27.2018) (28.994, -27.2692) knots 0 0 0 0 0.022562 0.043966 0.043966 0.043966 0.043966
  spline S85 degree 3 poles (28.994, -27.2692) (28.9654, -27.3287) (28.9119, -27.4405) (28.8206, -27.5241) (28.778, -27.5631) knots 0 0 0 0 0.019593 0.036773 0.036773 0.036773 0.036773
  spline S86 degree 3 poles (28.778, -27.5631) (28.7325, -27.5939) (28.6406, -27.6559) (28.534, -27.6864) (28.4801, -27.7018) knots 0 0 0 0 0.016361 0.033043 0.033043 0.033043 0.033043
  spline S87 degree 3 poles (28.4801, -27.7018) (28.4128, -27.7131) (28.255, -27.7396) (28.0948, -27.7402) (28.0031, -27.7406) knots 0 0 0 0 0.020465 0.04793 0.04793 0.04793 0.04793
  line L101 (28.0031, -27.7406) -> (26.3373, -27.7397)
  line L102 (29.0222, -19.2509) -> (29.0219, -19.9121)
  line L103 (29.0219, -19.9121) -> (28.6281, -19.9119)
  spline S88 degree 3 poles (28.6281, -19.9119) (28.6925, -19.9591) (28.8233, -20.055) (28.9114, -20.1913) (28.956, -20.2604) knots 0 0 0 0 0.023752 0.048209 0.048209 0.048209 0.048209
  spline S89 degree 3 poles (28.956, -20.2604) (28.9928, -20.3362) (29.0674, -20.4901) (29.0771, -20.6609) (29.082, -20.7475) knots 0 0 0 0 0.025016 0.050764 0.050764 0.050764 0.050764
  spline S90 degree 3 poles (29.082, -20.7475) (29.0658, -20.898) (29.0331, -21.2031) (28.8224, -21.4266) (28.7156, -21.5398) knots 0 0 0 0 0.044117 0.08946 0.08946 0.08946 0.08946
  spline S91 degree 3 poles (28.7156, -21.5398) (28.5741, -21.6346) (28.2668, -21.8403) (27.8959, -21.8563) (27.6958, -21.8649) knots 0 0 0 0 0.050137 0.108879 0.108879 0.108879 0.108879
  spline S92 degree 3 poles (27.6958, -21.8649) (27.4907, -21.8562) (27.1118, -21.8402) (26.7968, -21.6318) (26.6523, -21.5362) knots 0 0 0 0 0.060219 0.111249 0.111249 0.111249 0.111249
  spline S93 degree 3 poles (26.6523, -21.5362) (26.5438, -21.4224) (26.3305, -21.1987) (26.297, -20.8918) (26.2805, -20.741) knots 0 0 0 0 0.04578 0.089992 0.089992 0.089992 0.089992
  spline S94 degree 3 poles (26.2805, -20.741) (26.2838, -20.6695) (26.2903, -20.5302) (26.3432, -20.4013) (26.369, -20.3385) knots 0 0 0 0 0.021284 0.041488 0.041488 0.041488 0.041488
  spline S95 degree 3 poles (26.369, -20.3385) (26.4067, -20.2749) (26.4899, -20.1344) (26.6076, -20.021) (26.6721, -19.9588) knots 0 0 0 0 0.022061 0.048776 0.048776 0.048776 0.048776
  line L104 (26.6721, -19.9588) -> (25.3218, -19.9581)
  line L105 (25.3218, -19.9581) -> (25.3222, -19.2489)
  line L106 (25.3222, -19.2489) -> (29.0222, -19.2509)
  circle A8 centre (15, -30.5) radius 1.75
  circle A9 centre (15, -23.5) radius 1.75
  circle A10 centre (-15, -30.5) radius 1.75
  circle A11 centre (-15, -23.5) radius 1.75
  line L107 (15, -30.5) -> (15, -23.5) construction
  line L108 (-15, -30.5) -> (-15, -23.5) construction
  line L109 (15, -27) -> (-15, -27) construction
  line L110 (20, -19) -> (-20, -19)
  line L111 (-20, -19) -> (-20, -35)
  line L112 (-20, -35) -> (20, -35)
  line L113 (20, -35) -> (20, -19)
  line L114 (20, -19) -> (-20, -35) construction
  line L115 (-20, -19) -> (20, -35) construction
  line L116 (-10, -19) -> (10, -19)
  line L117 (10, -19) -> (10, -35)
  line L118 (10, -35) -> (-10, -35)
  line L119 (-10, -35) -> (-10, -19)
  line L120 (-10, -19) -> (10, -35) construction
  line L121 (10, -19) -> (-10, -35) construction
  line L122 (-4.5, -19) -> (4.5, -19)
  line L123 (4.5, -19) -> (4.5, -35)
  line L124 (4.5, -35) -> (-4.5, -35)
  line L125 (-4.5, -35) -> (-4.5, -19)
  line L126 (-4.5, -19) -> (4.5, -35) construction
  line L127 (4.5, -19) -> (-4.5, -35) construction
  line L128 (4.5, -29) -> (-4.5, -29)
  point P0 (0, -27)
  point P1 (0, -27)
  point P2 (0, -27)
  dimension "d94" = 40
  dimension "d95" = 16
  dimension "d96" = 20
  dimension "d97" = 9
  dimension "d105" = 10
  constraint midpoint L107 L109.start
  constraint midpoint L108 L109.end
  constraint horizontal L110
  constraint perpendicular L110 L111
  constraint parallel L110 L112
  constraint parallel L111 L113
  constraint coincident L114 P2
  constraint coincident L115 P2
  constraint midpoint L109 P2
  constraint horizontal L116
  constraint perpendicular L116 L117
  constraint parallel L116 L118
  constraint parallel L117 L119
  constraint coincident L120 P2
  constraint coincident L121 P2
  constraint coincident L110 L116.start
  constraint coincident P2 P1
  constraint horizontal L122
  constraint perpendicular L122 L123
  constraint parallel L122 L124
  constraint parallel L123 L125
  constraint coincident L126 P2
  constraint coincident L127 P2
  constraint coincident L116 L122.start
  constraint coincident L123 L128.start
  constraint coincident L125 L128.end
  constraint perpendicular L125 L128
  measures "d94" distance of L111.end L112.end
  measures "d95" distance of L110.end L111.end
  measures "d96" distance of L116.start L116.end
  measures "d97" distance of L123 L125
  measures "d105" distance of L110 L128
extrude "Extrude1''" add sketch "Sketch1 (2)" along normal blind 4 separate body contours L12 L25 L110 L111 L119 | L12 L35 L110 L113 L117 makes body 3 at (-11.0296, 25.9298, 6.5) makes body 4 at (11.0296, 25.9298, 6.5) in component "Weight mount"
extrude "Extrude3''" add sketch "Sketch1 (2)" along normal blind 16 contours L12 L25 L110 L116 L119 L125 | L12 L35 L110 L116 L117 L123 bodies 3 4 in component "Weight mount"
extrude "Extrude2''" add sketch "Sketch1 (2)" along normal up to surface (6.5 mm away) from surface at 9.5 contours L12 L123 L125 L128 | L25 L35 L110 L116 L122 L123 L125 L128 bodies 4 3 in component "Weight mount"
extrude "Extrude4'" cut sketch "Sketch1 (2)" along normal up to surface (16 mm away) contours L25 L35 L110 L116 L122 L123 L125 L128 bodies 4 in component "Weight mount"
sketch "Sketch3" plane through (10, 0, 0) normal (1, 0, 0) x (0, 1, 0) in component "Weight mount"
  line L0 (19, 10.5) -> (34.7, 10.5)
  line L1 (34.7, 10.5) -> (34.7, 22.5)
  line L2 (34.7, 22.5) -> (19, 22.5)
  line L3 (19, 22.5) -> (19, 10.5)
  line L4 (29, 16) -> (29, 22.5)
  line L5 (34.7, 16) -> (29, 16)
  circle A0 centre (24, 19.25) radius 1.75
  circle A1 centre (24, 19.25) radius 1.425
  circle A2 centre (24, 19.25) radius 2.575
  dimension "d108" = 3.5
  dimension "d109" = 2.85
  dimension "d110" = 5.15
  constraint concentric A0 A1
  constraint concentric A0 A2
  measures "d108" diameter of A0
  measures "d109" diameter of A1
  measures "d110" diameter of A2
extrude "Extrude5" cut sketch "Sketch3" against normal up to surface (20 mm away) contours A1 bodies 4 in component "Weight mount"
extrude "Extrude6" cut sketch "Sketch3" against normal up to surface (5.5 mm away) contours A0 bodies 4 in component "Weight mount"
extrude "Extrude7" cut sketch "Sketch3" against normal blind 2 contours A2 bodies 4 in component "Weight mount"
fillet "Fillet1''" radius 0.25 tangency weight 1.02347 1 edges at (-4.5, 22.6714, 19.7653) on bodies 4 in component "Weight mount"
fillet "Fillet1''" radius 0.15 1 edges at (8, 22.3684, 18.6172) on bodies 4 in component "Weight mount"
fillet "Fillet1''" radius 0.15 4 edges at (16.8647, 29.7768, 10.5) (16.8647, 22.7768, 10.5) (-13.1353, 22.7768, 10.5) (-13.1353, 29.7768, 10.5) on bodies 4 in component "Weight mount"
fillet "Fillet1''" radius 3.5 2 edges at (7.25, 19, 22.5) (-7.25, 19, 22.5) on bodies 4 in component "Weight mount"
fillet "Fillet1''" radius 1 1 edges at (0, 34.7, 22.5) on bodies 4 in component "Weight mount"
fillet "Fillet1''" radius 0.15 1 edges at (10, 21.5993, 20.1812) on bodies 4 in component "Weight mount"
chamfer "Chamfer1''" distance 0.5 angle 45 16 edges at (-10, 20.0251, 21.4749) (-10, 19, 14.75) (-10, 34.7, 16) (-10, 34.4071, 22.2071) (-10, 28.1, 22.5) (-15, 19, 10.5) (-20, 26.85, 10.5) (-15, 34.7, 10.5) (10, 19, 14.75) (10, 20.0251, 21.4749) (10, 28.1, 22.5) (10, 34.4071, 22.2071) (10, 34.7, 16) (15, 19, 10.5) (20, 26.85, 10.5) (15, 34.7, 10.5) on bodies 4 in component "Weight mount"
chamfer "Chamfer1''" distance 0.25 angle 45 7 edges at (-4.5, 19, 12.75) (-4.5, 20.0251, 21.4749) (-4.5, 25.75, 22.5) (0, 29, 22.5) (4.5, 20.0251, 21.4749) (4.5, 19, 12.75) (4.5, 25.75, 22.5) on bodies 4 in component "Weight mount"
component "Pen Mount" placed x (1, 0, 0) y (0, 1, 0) z (0, 0, 1) at (0, 0, 0)
component "Clamp" placed x (1, 0, 0) y (0, 1, 0) z (0, 0, 1) at (0, 0, 0)
component "Weight mount" placed x (1, 0, 0) y (0, 1, 0) z (0, 0, 1) at (0, 0, 0)
equation "d8 = flexure_thickness"
equation "d9 = flexure_thickness"
equation "flexure_thickness = 2 * nozzle_diameter"
equation "d12 = flexure_clearance_push"
equation "d13 = flexure_clearance_pull"
equation "d14 = flexure_clearance_pull"
equation "flexure_clearance_pull = 1 mm"
equation "d16 = flexure_clearance_pull"
equation "d17 = flexure_clearance_pull"
equation "d18 = flexure_clearance_pull"
equation "d20 = flexure_thickness"
equation "flexure_clearance_push = 6 mm"
equation "d22 = flexure_clearance_push"
equation "nozzle_diameter = 0.4 mm"
equation "d36 = mount_thickness"
equation "BIC_pen_diameter_max = 8.533 mm"
equation "d40 = ( BIC_pen_diameter_max / 2 )"
equation "d42 = ( BIC_pen_diameter_min / 2 ) - 0.0 mm"
equation "BIC_pen_diameter_min = 7.39 mm"
equation "d48 = ( BIC_pen_diameter_min / 2 ) - 0.7 mm"
equation "mount_thickness = 6.5 mm"
